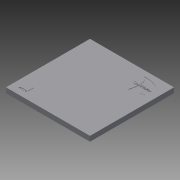
# Autodesk Inventor part: EmbossTest
Saved by Autodesk Inventor 2015 (Build 190159000, 159)
## iProperties
Created: 2014-08-09
Part Number: EmbossTest
Material: Generic
Document SubType Name: Modeling
Designer: Patrick Camilleri
Density: 1 g/cm^3
Appearance: Default
Author: Patrick Camilleri
Autodesk Inventor part; units mm, degrees
(part 1 of 2)
ref_plane "YZ Plane" through (0, 0, 0) normal (1, 0, 0) x (0, 1, 0)
ref_plane "XZ Plane" through (0, 0, 0) normal (0, 1, 0) x (-1, 0, 0)
ref_plane "XY Plane" through (0, 0, 0) normal (0, 0, 1) x (1, 0, 0)
sketch "Sketch1" plane through (0, 0, 0) normal (0, 0, 1) x (1, 0, 0)
  line L0 (-50, 50) -> (50, 50)
  line L1 (50, 50) -> (50, -50)
  line L2 (50, -50) -> (-50, -50)
  line L3 (-50, -50) -> (-50, 50)
  line L4 (-50, 50) -> (50, -50) construction
  line L5 (50, 50) -> (-50, -50) construction
  point P0 (0, 0)
  dimension "d0" = 100
  dimension "d1" = 100
  constraints: 12 end point, 2 midpoint, 2 parallel, 1 horizontal, 1 perpendicular
  measures "d0" distance of L1.end L2.end
  measures "d1" distance of L0.end L1.end
extrude "Extrusion1" add sketch "Sketch1" along normal blind 6
sketch "Sketch2" plane through (0, 0, 6) normal (0, 0, 1) x (1, 0, 0)
  spline S0 degree 3 poles (-34.8118, -41.5172) (-35.008, -41.7253) (-35.2042, -41.9334) (-35.4003, -42.1415) (-35.491, -42.2378) (-35.5355, -42.2383) (-35.6243, -42.1439) (-35.8031, -41.9538) (-35.9823, -41.7641) (-36.1607, -41.5736) (-36.1793, -41.5537) (-36.1936, -41.5297) (-36.2099, -41.5077) (-36.2185, -41.5128) (-36.2271, -41.5179) (-36.2357, -41.523) (-36.2357, -41.9827) (-36.2357, -42.4423) (-36.2357, -42.9059) (-36.4488, -42.9059) (-36.6508, -42.9059) (-36.8568, -42.9059) (-36.8568, -42.1529) (-36.8568, -41.4056) (-36.8568, -40.6466) (-36.6841, -40.6466) (-36.5132, -40.6444) (-36.3424, -40.649) (-36.3174, -40.6497) (-36.29, -40.6795) (-36.269, -40.701) (-36.0168, -40.9595) (-35.7656, -41.219) (-35.4885, -41.5046) (-35.4711, -41.4734) (-35.4606, -41.4412) (-35.4396, -41.4189) (-35.2133, -41.179) (-34.9844, -40.9416) (-34.7587, -40.701) (-34.7199, -40.6596) (-34.6805, -40.6436) (-34.6245, -40.6449) (-34.4757, -40.6483) (-34.3267, -40.646) (-34.1712, -40.646) (-34.1712, -41.4005) (-34.1712, -42.1498) (-34.1712, -42.9054) (-34.3761, -42.9054) (-34.5781, -42.9054) (-34.7897, -42.9054) (-34.7897, -42.4441) (-34.7897, -41.9842) (-34.7897, -41.5243) (-34.797, -41.522) (-34.8044, -41.5196) (-34.8118, -41.5172) knots 0 0 0 0 1 1 1 2 2 2 3 3 3 4 4 4 5 5 5 6 6 6 7 7 7 8 8 8 9 9 9 10 10 10 11 11 11 12 12 12 13 13 13 14 14 14 15 15 15 16 16 16 17 17 17 18 18 18 19 19 19 19
  line L0 (-34.8118, -41.5172) -> (-35.008, -41.7253) construction
  line L1 (-35.008, -41.7253) -> (-35.2042, -41.9334) construction
  line L2 (-35.2042, -41.9334) -> (-35.4003, -42.1415) construction
  line L3 (-35.4003, -42.1415) -> (-35.491, -42.2378) construction
  line L4 (-35.491, -42.2378) -> (-35.5355, -42.2383) construction
  line L5 (-35.5355, -42.2383) -> (-35.6243, -42.1439) construction
  line L6 (-35.6243, -42.1439) -> (-35.8031, -41.9538) construction
  line L7 (-35.8031, -41.9538) -> (-35.9823, -41.7641) construction
  line L8 (-35.9823, -41.7641) -> (-36.1607, -41.5736) construction
  line L9 (-36.1607, -41.5736) -> (-36.1793, -41.5537) construction
  line L10 (-36.1793, -41.5537) -> (-36.1936, -41.5297) construction
  line L11 (-36.1936, -41.5297) -> (-36.2099, -41.5077) construction
  line L12 (-36.2099, -41.5077) -> (-36.2185, -41.5128) construction
  line L13 (-36.2185, -41.5128) -> (-36.2271, -41.5179) construction
  line L14 (-36.2271, -41.5179) -> (-36.2357, -41.523) construction
  line L15 (-36.2357, -41.523) -> (-36.2357, -41.9827) construction
  line L16 (-36.2357, -41.9827) -> (-36.2357, -42.4423) construction
  line L17 (-36.2357, -42.4423) -> (-36.2357, -42.9059) construction
  line L18 (-36.2357, -42.9059) -> (-36.4488, -42.9059) construction
  line L19 (-36.4488, -42.9059) -> (-36.6508, -42.9059) construction
  line L20 (-36.6508, -42.9059) -> (-36.8568, -42.9059) construction
  line L21 (-36.8568, -42.9059) -> (-36.8568, -42.1529) construction
  line L22 (-36.8568, -42.1529) -> (-36.8568, -41.4056) construction
  line L23 (-36.8568, -41.4056) -> (-36.8568, -40.6466) construction
  line L24 (-36.8568, -40.6466) -> (-36.6841, -40.6466) construction
  line L25 (-36.6841, -40.6466) -> (-36.5132, -40.6444) construction
  line L26 (-36.5132, -40.6444) -> (-36.3424, -40.649) construction
  line L27 (-36.3424, -40.649) -> (-36.3174, -40.6497) construction
  line L28 (-36.3174, -40.6497) -> (-36.29, -40.6795) construction
  line L29 (-36.29, -40.6795) -> (-36.269, -40.701) construction
  line L30 (-36.269, -40.701) -> (-36.0168, -40.9595) construction
  line L31 (-36.0168, -40.9595) -> (-35.7656, -41.219) construction
  line L32 (-35.7656, -41.219) -> (-35.4885, -41.5046) construction
  line L33 (-35.4885, -41.5046) -> (-35.4711, -41.4734) construction
  line L34 (-35.4711, -41.4734) -> (-35.4606, -41.4412) construction
  line L35 (-35.4606, -41.4412) -> (-35.4396, -41.4189) construction
  line L36 (-35.4396, -41.4189) -> (-35.2133, -41.179) construction
  line L37 (-35.2133, -41.179) -> (-34.9844, -40.9416) construction
  line L38 (-34.9844, -40.9416) -> (-34.7587, -40.701) construction
  line L39 (-34.7587, -40.701) -> (-34.7199, -40.6596) construction
  line L40 (-34.7199, -40.6596) -> (-34.6805, -40.6436) construction
  line L41 (-34.6805, -40.6436) -> (-34.6245, -40.6449) construction
  line L42 (-34.6245, -40.6449) -> (-34.4757, -40.6483) construction
  line L43 (-34.4757, -40.6483) -> (-34.3267, -40.646) construction
  line L44 (-34.3267, -40.646) -> (-34.1712, -40.646) construction
  line L45 (-34.1712, -40.646) -> (-34.1712, -41.4005) construction
  line L46 (-34.1712, -41.4005) -> (-34.1712, -42.1498) construction
  line L47 (-34.1712, -42.1498) -> (-34.1712, -42.9054) construction
  line L48 (-34.1712, -42.9054) -> (-34.3761, -42.9054) construction
  line L49 (-34.3761, -42.9054) -> (-34.5781, -42.9054) construction
  line L50 (-34.5781, -42.9054) -> (-34.7897, -42.9054) construction
  line L51 (-34.7897, -42.9054) -> (-34.7897, -42.4441) construction
  line L52 (-34.7897, -42.4441) -> (-34.7897, -41.9842) construction
  line L53 (-34.7897, -41.9842) -> (-34.7897, -41.5243) construction
  line L54 (-34.7897, -41.5243) -> (-34.797, -41.522) construction
  line L55 (-34.797, -41.522) -> (-34.8044, -41.5196) construction
  line L56 (-34.8044, -41.5196) -> (-34.8118, -41.5172) construction
  spline S1 degree 3 poles (-39.2287, -40.6616) (-38.7914, -40.6616) (-38.3614, -40.6502) (-37.9325, -40.6665) (-37.7171, -40.6747) (-37.5328, -40.7855) (-37.4045, -40.9677) (-37.2119, -41.2411) (-37.2808, -41.5889) (-37.5615, -41.7698) (-37.6066, -41.7989) (-37.6545, -41.8234) (-37.709, -41.8545) (-37.5451, -41.9467) (-37.4576, -42.0939) (-37.3778, -42.2464) (-37.2652, -42.4612) (-37.1555, -42.6775) (-37.0396, -42.9027) (-37.073, -42.9065) (-37.0944, -42.9111) (-37.1158, -42.9112) (-37.2936, -42.9118) (-37.4714, -42.9093) (-37.6491, -42.9128) (-37.703, -42.9139) (-37.7326, -42.8953) (-37.7552, -42.8482) (-37.8172, -42.7192) (-37.8821, -42.5916) (-37.9469, -42.464) (-37.9819, -42.3951) (-38.0185, -42.3269) (-38.0554, -42.259) (-38.1716, -42.0454) (-38.3477, -41.9527) (-38.601, -41.9994) (-38.6025, -42.0249) (-38.6059, -42.0549) (-38.606, -42.085) (-38.6064, -42.3344) (-38.6078, -42.5839) (-38.6051, -42.8333) (-38.6045, -42.8918) (-38.6202, -42.914) (-38.682, -42.9127) (-38.862, -42.9092) (-39.0422, -42.9115) (-39.2287, -42.9115) (-39.2287, -42.1545) (-39.2287, -41.4055) (-39.2287, -40.6616) knots 0 0 0 0 1 1 1 2 2 2 3 3 3 4 4 4 5 5 5 6 6 6 7 7 7 8 8 8 9 9 9 10 10 10 11 11 11 12 12 12 13 13 13 14 14 14 15 15 15 16 16 16 17 17 17 17
  line L57 (-39.2287, -40.6616) -> (-38.7914, -40.6616) construction
  line L58 (-38.7914, -40.6616) -> (-38.3614, -40.6502) construction
  line L59 (-38.3614, -40.6502) -> (-37.9325, -40.6665) construction
  line L60 (-37.9325, -40.6665) -> (-37.7171, -40.6747) construction
  line L61 (-37.7171, -40.6747) -> (-37.5328, -40.7855) construction
  line L62 (-37.5328, -40.7855) -> (-37.4045, -40.9677) construction
  line L63 (-37.4045, -40.9677) -> (-37.2119, -41.2411) construction
  line L64 (-37.2119, -41.2411) -> (-37.2808, -41.5889) construction
  line L65 (-37.2808, -41.5889) -> (-37.5615, -41.7698) construction
  line L66 (-37.5615, -41.7698) -> (-37.6066, -41.7989) construction
  line L67 (-37.6066, -41.7989) -> (-37.6545, -41.8234) construction
  line L68 (-37.6545, -41.8234) -> (-37.709, -41.8545) construction
  line L69 (-37.709, -41.8545) -> (-37.5451, -41.9467) construction
  line L70 (-37.5451, -41.9467) -> (-37.4576, -42.0939) construction
  line L71 (-37.4576, -42.0939) -> (-37.3778, -42.2464) construction
  line L72 (-37.3778, -42.2464) -> (-37.2652, -42.4612) construction
  line L73 (-37.2652, -42.4612) -> (-37.1555, -42.6775) construction
  line L74 (-37.1555, -42.6775) -> (-37.0396, -42.9027) construction
  line L75 (-37.0396, -42.9027) -> (-37.073, -42.9065) construction
  line L76 (-37.073, -42.9065) -> (-37.0944, -42.9111) construction
  line L77 (-37.0944, -42.9111) -> (-37.1158, -42.9112) construction
  line L78 (-37.1158, -42.9112) -> (-37.2936, -42.9118) construction
  line L79 (-37.2936, -42.9118) -> (-37.4714, -42.9093) construction
  line L80 (-37.4714, -42.9093) -> (-37.6491, -42.9128) construction
  line L81 (-37.6491, -42.9128) -> (-37.703, -42.9139) construction
  line L82 (-37.703, -42.9139) -> (-37.7326, -42.8953) construction
  line L83 (-37.7326, -42.8953) -> (-37.7552, -42.8482) construction
  line L84 (-37.7552, -42.8482) -> (-37.8172, -42.7192) construction
  line L85 (-37.8172, -42.7192) -> (-37.8821, -42.5916) construction
  line L86 (-37.8821, -42.5916) -> (-37.9469, -42.464) construction
  line L87 (-37.9469, -42.464) -> (-37.9819, -42.3951) construction
  line L88 (-37.9819, -42.3951) -> (-38.0185, -42.3269) construction
  line L89 (-38.0185, -42.3269) -> (-38.0554, -42.259) construction
  line L90 (-38.0554, -42.259) -> (-38.1716, -42.0454) construction
  line L91 (-38.1716, -42.0454) -> (-38.3477, -41.9527) construction
  line L92 (-38.3477, -41.9527) -> (-38.601, -41.9994) construction
  line L93 (-38.601, -41.9994) -> (-38.6025, -42.0249) construction
  line L94 (-38.6025, -42.0249) -> (-38.6059, -42.0549) construction
  line L95 (-38.6059, -42.0549) -> (-38.606, -42.085) construction
  line L96 (-38.606, -42.085) -> (-38.6064, -42.3344) construction
  line L97 (-38.6064, -42.3344) -> (-38.6078, -42.5839) construction
  line L98 (-38.6078, -42.5839) -> (-38.6051, -42.8333) construction
  line L99 (-38.6051, -42.8333) -> (-38.6045, -42.8918) construction
  line L100 (-38.6045, -42.8918) -> (-38.6202, -42.914) construction
  line L101 (-38.6202, -42.914) -> (-38.682, -42.9127) construction
  line L102 (-38.682, -42.9127) -> (-38.862, -42.9092) construction
  line L103 (-38.862, -42.9092) -> (-39.0422, -42.9115) construction
  line L104 (-39.0422, -42.9115) -> (-39.2287, -42.9115) construction
  line L105 (-39.2287, -42.9115) -> (-39.2287, -42.1545) construction
  line L106 (-39.2287, -42.1545) -> (-39.2287, -41.4055) construction
  line L107 (-39.2287, -41.4055) -> (-39.2287, -40.6616) construction
  spline S2 degree 3 poles (-38.6, -41.0537) (-38.6, -41.2363) (-38.6, -41.4025) (-38.6, -41.5842) (-38.4373, -41.5746) (-38.2798, -41.5763) (-38.1261, -41.553) (-37.9994, -41.5338) (-37.9376, -41.4371) (-37.9393, -41.3124) (-37.9411, -41.1891) (-38.0091, -41.0963) (-38.1362, -41.0804) (-38.2878, -41.0614) (-38.4418, -41.0619) (-38.6, -41.0537) knots 0 0 0 0 1 1 1 2 2 2 3 3 3 4 4 4 5 5 5 5
  line L108 (-38.6, -41.0537) -> (-38.6, -41.2363) construction
  line L109 (-38.6, -41.2363) -> (-38.6, -41.4025) construction
  line L110 (-38.6, -41.4025) -> (-38.6, -41.5842) construction
  line L111 (-38.6, -41.5842) -> (-38.4373, -41.5746) construction
  line L112 (-38.4373, -41.5746) -> (-38.2798, -41.5763) construction
  line L113 (-38.2798, -41.5763) -> (-38.1261, -41.553) construction
  line L114 (-38.1261, -41.553) -> (-37.9994, -41.5338) construction
  line L115 (-37.9994, -41.5338) -> (-37.9376, -41.4371) construction
  line L116 (-37.9376, -41.4371) -> (-37.9393, -41.3124) construction
  line L117 (-37.9393, -41.3124) -> (-37.9411, -41.1891) construction
  line L118 (-37.9411, -41.1891) -> (-38.0091, -41.0963) construction
  line L119 (-38.0091, -41.0963) -> (-38.1362, -41.0804) construction
  line L120 (-38.1362, -41.0804) -> (-38.2878, -41.0614) construction
  line L121 (-38.2878, -41.0614) -> (-38.4418, -41.0619) construction
  line L122 (-38.4418, -41.0619) -> (-38.6, -41.0537) construction
  spline S3 degree 3 poles (-39.3868, -42.9109) (-39.605, -42.9109) (-39.813, -42.9124) (-40.0209, -42.9084) (-40.0397, -42.908) (-40.0643, -42.8756) (-40.0752, -42.8528) (-40.126, -42.7469) (-40.1755, -42.6404) (-40.22, -42.5319) (-40.2419, -42.4784) (-40.2731, -42.4621) (-40.3302, -42.4626) (-40.6513, -42.4656) (-40.9724, -42.4654) (-41.2935, -42.4629) (-41.3528, -42.4624) (-41.3864, -42.4767) (-41.408, -42.5368) (-41.4466, -42.6444) (-41.4937, -42.7491) (-41.5418, -42.8529) (-41.5528, -42.8767) (-41.5817, -42.9083) (-41.6029, -42.9088) (-41.8028, -42.913) (-42.0029, -42.9113) (-42.2145, -42.9113) (-42.1997, -42.873) (-42.1901, -42.8444) (-42.1779, -42.817) (-41.8681, -42.1183) (-41.5576, -41.42) (-41.2493, -40.7208) (-41.2256, -40.6671) (-41.1998, -40.6427) (-41.1367, -40.6443) (-40.9419, -40.6492) (-40.7468, -40.6473) (-40.5519, -40.6451) (-40.5067, -40.6447) (-40.4803, -40.6557) (-40.4591, -40.6996) (-40.11, -41.4179) (-39.7589, -42.1353) (-39.4085, -42.853) (-39.4015, -42.8675) (-39.3971, -42.8832) (-39.3868, -42.9109) knots 0 0 0 0 1 1 1 2 2 2 3 3 3 4 4 4 5 5 5 6 6 6 7 7 7 8 8 8 9 9 9 10 10 10 11 11 11 12 12 12 13 13 13 14 14 14 15 15 15 16 16 16 16
  line L123 (-39.3868, -42.9109) -> (-39.605, -42.9109) construction
  line L124 (-39.605, -42.9109) -> (-39.813, -42.9124) construction
  line L125 (-39.813, -42.9124) -> (-40.0209, -42.9084) construction
  line L126 (-40.0209, -42.9084) -> (-40.0397, -42.908) construction
  line L127 (-40.0397, -42.908) -> (-40.0643, -42.8756) construction
  line L128 (-40.0643, -42.8756) -> (-40.0752, -42.8528) construction
  line L129 (-40.0752, -42.8528) -> (-40.126, -42.7469) construction
  line L130 (-40.126, -42.7469) -> (-40.1755, -42.6404) construction
  line L131 (-40.1755, -42.6404) -> (-40.22, -42.5319) construction
  line L132 (-40.22, -42.5319) -> (-40.2419, -42.4784) construction
  line L133 (-40.2419, -42.4784) -> (-40.2731, -42.4621) construction
  line L134 (-40.2731, -42.4621) -> (-40.3302, -42.4626) construction
  line L135 (-40.3302, -42.4626) -> (-40.6513, -42.4656) construction
  line L136 (-40.6513, -42.4656) -> (-40.9724, -42.4654) construction
  line L137 (-40.9724, -42.4654) -> (-41.2935, -42.4629) construction
  line L138 (-41.2935, -42.4629) -> (-41.3528, -42.4624) construction
  line L139 (-41.3528, -42.4624) -> (-41.3864, -42.4767) construction
  line L140 (-41.3864, -42.4767) -> (-41.408, -42.5368) construction
  line L141 (-41.408, -42.5368) -> (-41.4466, -42.6444) construction
  line L142 (-41.4466, -42.6444) -> (-41.4937, -42.7491) construction
  line L143 (-41.4937, -42.7491) -> (-41.5418, -42.8529) construction
  line L144 (-41.5418, -42.8529) -> (-41.5528, -42.8767) construction
  line L145 (-41.5528, -42.8767) -> (-41.5817, -42.9083) construction
  line L146 (-41.5817, -42.9083) -> (-41.6029, -42.9088) construction
  line L147 (-41.6029, -42.9088) -> (-41.8028, -42.913) construction
  line L148 (-41.8028, -42.913) -> (-42.0029, -42.9113) construction
  line L149 (-42.0029, -42.9113) -> (-42.2145, -42.9113) construction
  line L150 (-42.2145, -42.9113) -> (-42.1997, -42.873) construction
  line L151 (-42.1997, -42.873) -> (-42.1901, -42.8444) construction
  line L152 (-42.1901, -42.8444) -> (-42.1779, -42.817) construction
  line L153 (-42.1779, -42.817) -> (-41.8681, -42.1183) construction
  line L154 (-41.8681, -42.1183) -> (-41.5576, -41.42) construction
  line L155 (-41.5576, -41.42) -> (-41.2493, -40.7208) construction
  line L156 (-41.2493, -40.7208) -> (-41.2256, -40.6671) construction
  line L157 (-41.2256, -40.6671) -> (-41.1998, -40.6427) construction
  line L158 (-41.1998, -40.6427) -> (-41.1367, -40.6443) construction
  line L159 (-41.1367, -40.6443) -> (-40.9419, -40.6492) construction
  line L160 (-40.9419, -40.6492) -> (-40.7468, -40.6473) construction
  line L161 (-40.7468, -40.6473) -> (-40.5519, -40.6451) construction
  line L162 (-40.5519, -40.6451) -> (-40.5067, -40.6447) construction
  line L163 (-40.5067, -40.6447) -> (-40.4803, -40.6557) construction
  line L164 (-40.4803, -40.6557) -> (-40.4591, -40.6996) construction
  line L165 (-40.4591, -40.6996) -> (-40.11, -41.4179) construction
  line L166 (-40.11, -41.4179) -> (-39.7589, -42.1353) construction
  line L167 (-39.7589, -42.1353) -> (-39.4085, -42.853) construction
  line L168 (-39.4085, -42.853) -> (-39.4015, -42.8675) construction
  line L169 (-39.4015, -42.8675) -> (-39.3971, -42.8832) construction
  line L170 (-39.3971, -42.8832) -> (-39.3868, -42.9109) construction
  spline S4 degree 3 poles (-40.8503, -41.1882) (-40.9747, -41.4892) (-41.0919, -41.7726) (-41.2123, -42.0639) (-40.9517, -42.0639) (-40.7052, -42.0639) (-40.4452, -42.0639) (-40.5801, -41.7725) (-40.7104, -41.4908) (-40.8503, -41.1882) knots 0 0 0 0 1 1 1 2 2 2 3 3 3 3
  line L171 (-40.8503, -41.1882) -> (-40.9747, -41.4892) construction
  line L172 (-40.9747, -41.4892) -> (-41.0919, -41.7726) construction
  line L173 (-41.0919, -41.7726) -> (-41.2123, -42.0639) construction
  line L174 (-41.2123, -42.0639) -> (-40.9517, -42.0639) construction
  line L175 (-40.9517, -42.0639) -> (-40.7052, -42.0639) construction
  line L176 (-40.7052, -42.0639) -> (-40.4452, -42.0639) construction
  line L177 (-40.4452, -42.0639) -> (-40.5801, -41.7725) construction
  line L178 (-40.5801, -41.7725) -> (-40.7104, -41.4908) construction
  line L179 (-40.7104, -41.4908) -> (-40.8503, -41.1882) construction
  spline S5 degree 3 poles (-33.8681, -41.7853) (-33.4616, -41.7853) (-33.0617, -41.7853) (-32.6568, -41.7853) (-32.6568, -42.1521) (-32.6568, -42.5147) (-32.6568, -42.8858) (-33.0581, -42.8858) (-33.4597, -42.8858) (-33.8681, -42.8858) (-33.8681, -42.5215) (-33.8681, -42.1567) (-33.8681, -41.7853) knots 0 0 0 0 1 1 1 2 2 2 3 3 3 4 4 4 4
  line L180 (-33.8681, -41.7853) -> (-33.4616, -41.7853) construction
  line L181 (-33.4616, -41.7853) -> (-33.0617, -41.7853) construction
  line L182 (-33.0617, -41.7853) -> (-32.6568, -41.7853) construction
  line L183 (-32.6568, -41.7853) -> (-32.6568, -42.1521) construction
  line L184 (-32.6568, -42.1521) -> (-32.6568, -42.5147) construction
  line L185 (-32.6568, -42.5147) -> (-32.6568, -42.8858) construction
  line L186 (-32.6568, -42.8858) -> (-33.0581, -42.8858) construction
  line L187 (-33.0581, -42.8858) -> (-33.4597, -42.8858) construction
  line L188 (-33.4597, -42.8858) -> (-33.8681, -42.8858) construction
  line L189 (-33.8681, -42.8858) -> (-33.8681, -42.5215) construction
  line L190 (-33.8681, -42.5215) -> (-33.8681, -42.1567) construction
  line L191 (-33.8681, -42.1567) -> (-33.8681, -41.7853) construction
  spline S6 degree 3 poles (-33.7217, -38.9912) (-33.7217, -38.9387) (-33.7217, -38.8916) (-33.7217, -38.8362) (-33.3924, -38.7709) (-33.0623, -38.7054) (-32.7322, -38.64) (-32.7316, -38.6337) (-32.731, -38.6274) (-32.7304, -38.6211) (-32.8416, -38.5965) (-32.9527, -38.5713) (-33.0641, -38.5474) (-33.2515, -38.507) (-33.4382, -38.4621) (-33.6271, -38.4302) (-33.7109, -38.416) (-33.7412, -38.3833) (-33.728, -38.3024) (-33.724, -38.2775) (-33.7274, -38.2514) (-33.7274, -38.2181) (-33.3898, -38.1562) (-33.0567, -38.095) (-32.7235, -38.0338) (-32.7237, -38.0281) (-32.7239, -38.0224) (-32.7241, -38.0166) (-33.0236, -37.9482) (-33.3232, -37.88) (-33.6227, -37.8113) (-33.7406, -37.7842) (-33.7404, -37.7836) (-33.7165, -37.6482) (-33.5086, -37.7002) (-33.3012, -37.7521) (-33.0938, -37.8038) (-32.9245, -37.8459) (-32.7559, -37.8916) (-32.5852, -37.9279) (-32.5122, -37.9435) (-32.5195, -37.9881) (-32.5163, -38.0407) (-32.5128, -38.099) (-32.5415, -38.1107) (-32.5906, -38.1201) (-32.897, -38.1788) (-33.2027, -38.2407) (-33.5087, -38.3017) (-33.5236, -38.3047) (-33.5381, -38.3095) (-33.553, -38.3306) (-33.2108, -38.4036) (-32.8687, -38.4766) (-32.5301, -38.5489) (-32.5251, -38.5595) (-32.5211, -38.5644) (-32.5205, -38.5698) (-32.5041, -38.7211) (-32.5042, -38.7208) (-32.6525, -38.7541) (-32.9932, -38.8305) (-33.3338, -38.9071) (-33.6745, -38.9835) (-33.6879, -38.9865) (-33.7017, -38.988) (-33.7217, -38.9912) knots 0 0 0 0 1 1 1 2 2 2 3 3 3 4 4 4 5 5 5 6 6 6 7 7 7 8 8 8 9 9 9 10 10 10 11 11 11 12 12 12 13 13 13 14 14 14 15 15 15 16 16 16 17 17 17 18 18 18 19 19 19 20 20 20 21 21 21 22 22 22 22
  line L192 (-33.7217, -38.9912) -> (-33.7217, -38.9387) construction
  line L193 (-33.7217, -38.9387) -> (-33.7217, -38.8916) construction
  line L194 (-33.7217, -38.8916) -> (-33.7217, -38.8362) construction
  line L195 (-33.7217, -38.8362) -> (-33.3924, -38.7709) construction
  line L196 (-33.3924, -38.7709) -> (-33.0623, -38.7054) construction
  line L197 (-33.0623, -38.7054) -> (-32.7322, -38.64) construction
  line L198 (-32.7322, -38.64) -> (-32.7316, -38.6337) construction
  line L199 (-32.7316, -38.6337) -> (-32.731, -38.6274) construction
  line L200 (-32.731, -38.6274) -> (-32.7304, -38.6211) construction
  line L201 (-32.7304, -38.6211) -> (-32.8416, -38.5965) construction
  line L202 (-32.8416, -38.5965) -> (-32.9527, -38.5713) construction
  line L203 (-32.9527, -38.5713) -> (-33.0641, -38.5474) construction
  line L204 (-33.0641, -38.5474) -> (-33.2515, -38.507) construction
  line L205 (-33.2515, -38.507) -> (-33.4382, -38.4621) construction
  line L206 (-33.4382, -38.4621) -> (-33.6271, -38.4302) construction
  line L207 (-33.6271, -38.4302) -> (-33.7109, -38.416) construction
  line L208 (-33.7109, -38.416) -> (-33.7412, -38.3833) construction
  line L209 (-33.7412, -38.3833) -> (-33.728, -38.3024) construction
  line L210 (-33.728, -38.3024) -> (-33.724, -38.2775) construction
  line L211 (-33.724, -38.2775) -> (-33.7274, -38.2514) construction
  line L212 (-33.7274, -38.2514) -> (-33.7274, -38.2181) construction
  line L213 (-33.7274, -38.2181) -> (-33.3898, -38.1562) construction
  line L214 (-33.3898, -38.1562) -> (-33.0567, -38.095) construction
  line L215 (-33.0567, -38.095) -> (-32.7235, -38.0338) construction
  line L216 (-32.7235, -38.0338) -> (-32.7237, -38.0281) construction
  line L217 (-32.7237, -38.0281) -> (-32.7239, -38.0224) construction
  line L218 (-32.7239, -38.0224) -> (-32.7241, -38.0166) construction
  line L219 (-32.7241, -38.0166) -> (-33.0236, -37.9482) construction
  line L220 (-33.0236, -37.9482) -> (-33.3232, -37.88) construction
  line L221 (-33.3232, -37.88) -> (-33.6227, -37.8113) construction
  line L222 (-33.6227, -37.8113) -> (-33.7406, -37.7842) construction
  line L223 (-33.7406, -37.7842) -> (-33.7404, -37.7836) construction
  line L224 (-33.7404, -37.7836) -> (-33.7165, -37.6482) construction
  line L225 (-33.7165, -37.6482) -> (-33.5086, -37.7002) construction
  line L226 (-33.5086, -37.7002) -> (-33.3012, -37.7521) construction
  line L227 (-33.3012, -37.7521) -> (-33.0938, -37.8038) construction
  line L228 (-33.0938, -37.8038) -> (-32.9245, -37.8459) construction
  line L229 (-32.9245, -37.8459) -> (-32.7559, -37.8916) construction
  line L230 (-32.7559, -37.8916) -> (-32.5852, -37.9279) construction
  line L231 (-32.5852, -37.9279) -> (-32.5122, -37.9435) construction
  line L232 (-32.5122, -37.9435) -> (-32.5195, -37.9881) construction
  line L233 (-32.5195, -37.9881) -> (-32.5163, -38.0407) construction
  line L234 (-32.5163, -38.0407) -> (-32.5128, -38.099) construction
  line L235 (-32.5128, -38.099) -> (-32.5415, -38.1107) construction
  line L236 (-32.5415, -38.1107) -> (-32.5906, -38.1201) construction
  line L237 (-32.5906, -38.1201) -> (-32.897, -38.1788) construction
  line L238 (-32.897, -38.1788) -> (-33.2027, -38.2407) construction
  line L239 (-33.2027, -38.2407) -> (-33.5087, -38.3017) construction
  line L240 (-33.5087, -38.3017) -> (-33.5236, -38.3047) construction
  line L241 (-33.5236, -38.3047) -> (-33.5381, -38.3095) construction
  line L242 (-33.5381, -38.3095) -> (-33.553, -38.3306) construction
  line L243 (-33.553, -38.3306) -> (-33.2108, -38.4036) construction
  line L244 (-33.2108, -38.4036) -> (-32.8687, -38.4766) construction
  line L245 (-32.8687, -38.4766) -> (-32.5301, -38.5489) construction
  line L246 (-32.5301, -38.5489) -> (-32.5251, -38.5595) construction
  line L247 (-32.5251, -38.5595) -> (-32.5211, -38.5644) construction
  line L248 (-32.5211, -38.5644) -> (-32.5205, -38.5698) construction
  line L249 (-32.5205, -38.5698) -> (-32.5041, -38.7211) construction
  line L250 (-32.5041, -38.7211) -> (-32.5042, -38.7208) construction
  line L251 (-32.5042, -38.7208) -> (-32.6525, -38.7541) construction
  line L252 (-32.6525, -38.7541) -> (-32.9932, -38.8305) construction
  line L253 (-32.9932, -38.8305) -> (-33.3338, -38.9071) construction
  line L254 (-33.3338, -38.9071) -> (-33.6745, -38.9835) construction
  line L255 (-33.6745, -38.9835) -> (-33.6879, -38.9865) construction
  line L256 (-33.6879, -38.9865) -> (-33.7017, -38.988) construction
  line L257 (-33.7017, -38.988) -> (-33.7217, -38.9912) construction
  spline S7 degree 3 poles (-33.7147, -35.2257) (-33.7147, -35.0772) (-33.7216, -34.9371) (-33.7126, -34.7981) (-33.7053, -34.6847) (-33.6212, -34.6185) (-33.5216, -34.5885) (-33.3183, -34.5272) (-33.1082, -34.545) (-32.8999, -34.5575) (-32.8439, -34.5609) (-32.7864, -34.5714) (-32.7335, -34.5897) (-32.5911, -34.6387) (-32.5181, -34.7452) (-32.5179, -34.8936) (-32.5177, -34.9968) (-32.5186, -35.1) (-32.5194, -35.2033) (-32.5194, -35.2085) (-32.5232, -35.2138) (-32.5279, -35.2257) (-32.922, -35.2257) (-33.3187, -35.2257) (-33.7147, -35.2257) knots 0 0 0 0 1 1 1 2 2 2 3 3 3 4 4 4 5 5 5 6 6 6 7 7 7 8 8 8 8
  line L258 (-33.7147, -35.2257) -> (-33.7147, -35.0772) construction
  line L259 (-33.7147, -35.0772) -> (-33.7216, -34.9371) construction
  line L260 (-33.7216, -34.9371) -> (-33.7126, -34.7981) construction
  line L261 (-33.7126, -34.7981) -> (-33.7053, -34.6847) construction
  line L262 (-33.7053, -34.6847) -> (-33.6212, -34.6185) construction
  line L263 (-33.6212, -34.6185) -> (-33.5216, -34.5885) construction
  line L264 (-33.5216, -34.5885) -> (-33.3183, -34.5272) construction
  line L265 (-33.3183, -34.5272) -> (-33.1082, -34.545) construction
  line L266 (-33.1082, -34.545) -> (-32.8999, -34.5575) construction
  line L267 (-32.8999, -34.5575) -> (-32.8439, -34.5609) construction
  line L268 (-32.8439, -34.5609) -> (-32.7864, -34.5714) construction
  line L269 (-32.7864, -34.5714) -> (-32.7335, -34.5897) construction
  line L270 (-32.7335, -34.5897) -> (-32.5911, -34.6387) construction
  line L271 (-32.5911, -34.6387) -> (-32.5181, -34.7452) construction
  line L272 (-32.5181, -34.7452) -> (-32.5179, -34.8936) construction
  line L273 (-32.5179, -34.8936) -> (-32.5177, -34.9968) construction
  line L274 (-32.5177, -34.9968) -> (-32.5186, -35.1) construction
  line L275 (-32.5186, -35.1) -> (-32.5194, -35.2033) construction
  line L276 (-32.5194, -35.2033) -> (-32.5194, -35.2085) construction
  line L277 (-32.5194, -35.2085) -> (-32.5232, -35.2138) construction
  line L278 (-32.5232, -35.2138) -> (-32.5279, -35.2257) construction
  line L279 (-32.5279, -35.2257) -> (-32.922, -35.2257) construction
  line L280 (-32.922, -35.2257) -> (-33.3187, -35.2257) construction
  line L281 (-33.3187, -35.2257) -> (-33.7147, -35.2257) construction
  spline S8 degree 3 poles (-32.6481, -35.0843) (-32.6481, -35.0388) (-32.6499, -35.0019) (-32.6478, -34.9651) (-32.6391, -34.8163) (-32.7076, -34.7085) (-32.8525, -34.7051) (-33.0483, -34.7005) (-33.2448, -34.6987) (-33.4401, -34.7112) (-33.5222, -34.7164) (-33.5858, -34.7798) (-33.5945, -34.8708) (-33.6011, -34.9405) (-33.5958, -35.0114) (-33.5958, -35.0843) (-33.2779, -35.0843) (-32.9693, -35.0843) (-32.6481, -35.0843) knots 0 0 0 0 1 1 1 2 2 2 3 3 3 4 4 4 5 5 5 6 6 6 6
  line L282 (-32.6481, -35.0843) -> (-32.6481, -35.0388) construction
  line L283 (-32.6481, -35.0388) -> (-32.6499, -35.0019) construction
  line L284 (-32.6499, -35.0019) -> (-32.6478, -34.9651) construction
  line L285 (-32.6478, -34.9651) -> (-32.6391, -34.8163) construction
  line L286 (-32.6391, -34.8163) -> (-32.7076, -34.7085) construction
  line L287 (-32.7076, -34.7085) -> (-32.8525, -34.7051) construction
  line L288 (-32.8525, -34.7051) -> (-33.0483, -34.7005) construction
  line L289 (-33.0483, -34.7005) -> (-33.2448, -34.6987) construction
  line L290 (-33.2448, -34.6987) -> (-33.4401, -34.7112) construction
  line L291 (-33.4401, -34.7112) -> (-33.5222, -34.7164) construction
  line L292 (-33.5222, -34.7164) -> (-33.5858, -34.7798) construction
  line L293 (-33.5858, -34.7798) -> (-33.5945, -34.8708) construction
  line L294 (-33.5945, -34.8708) -> (-33.6011, -34.9405) construction
  line L295 (-33.6011, -34.9405) -> (-33.5958, -35.0114) construction
  line L296 (-33.5958, -35.0114) -> (-33.5958, -35.0843) construction
  line L297 (-33.5958, -35.0843) -> (-33.2779, -35.0843) construction
  line L298 (-33.2779, -35.0843) -> (-32.9693, -35.0843) construction
  line L299 (-32.9693, -35.0843) -> (-32.6481, -35.0843) construction
  spline S9 degree 3 poles (-32.5242, -36.1511) (-32.5077, -36.3021) (-32.5077, -36.3014) (-32.6514, -36.3105) (-32.7453, -36.3164) (-32.8401, -36.3187) (-32.9327, -36.3333) (-33.0313, -36.3489) (-33.0732, -36.4053) (-33.076, -36.5048) (-33.0774, -36.5529) (-33.0763, -36.6009) (-33.0763, -36.6593) (-32.8882, -36.6593) (-32.7089, -36.6593) (-32.5238, -36.6593) (-32.5238, -36.7109) (-32.5238, -36.7522) (-32.5238, -36.7992) (-32.923, -36.7992) (-33.3197, -36.7992) (-33.7249, -36.7992) (-33.7249, -36.6543) (-33.732, -36.5112) (-33.7224, -36.3693) (-33.7156, -36.2697) (-33.6217, -36.189) (-33.5261, -36.1683) (-33.3919, -36.1394) (-33.2722, -36.1529) (-33.183, -36.2707) (-33.1692, -36.2888) (-33.159, -36.3096) (-33.1416, -36.3382) (-33.1078, -36.2014) (-33.0053, -36.1892) (-32.8935, -36.184) (-32.7719, -36.1782) (-32.6509, -36.1628) (-32.5242, -36.1511) knots 0 0 0 0 1 1 1 2 2 2 3 3 3 4 4 4 5 5 5 6 6 6 7 7 7 8 8 8 9 9 9 10 10 10 11 11 11 12 12 12 13 13 13 13
  line L300 (-32.5242, -36.1511) -> (-32.5077, -36.3021) construction
  line L301 (-32.5077, -36.3021) -> (-32.5077, -36.3014) construction
  line L302 (-32.5077, -36.3014) -> (-32.6514, -36.3105) construction
  line L303 (-32.6514, -36.3105) -> (-32.7453, -36.3164) construction
  line L304 (-32.7453, -36.3164) -> (-32.8401, -36.3187) construction
  line L305 (-32.8401, -36.3187) -> (-32.9327, -36.3333) construction
  line L306 (-32.9327, -36.3333) -> (-33.0313, -36.3489) construction
  line L307 (-33.0313, -36.3489) -> (-33.0732, -36.4053) construction
  line L308 (-33.0732, -36.4053) -> (-33.076, -36.5048) construction
  line L309 (-33.076, -36.5048) -> (-33.0774, -36.5529) construction
  line L310 (-33.0774, -36.5529) -> (-33.0763, -36.6009) construction
  line L311 (-33.0763, -36.6009) -> (-33.0763, -36.6593) construction
  line L312 (-33.0763, -36.6593) -> (-32.8882, -36.6593) construction
  line L313 (-32.8882, -36.6593) -> (-32.7089, -36.6593) construction
  line L314 (-32.7089, -36.6593) -> (-32.5238, -36.6593) construction
  line L315 (-32.5238, -36.6593) -> (-32.5238, -36.7109) construction
  line L316 (-32.5238, -36.7109) -> (-32.5238, -36.7522) construction
  line L317 (-32.5238, -36.7522) -> (-32.5238, -36.7992) construction
  line L318 (-32.5238, -36.7992) -> (-32.923, -36.7992) construction
  line L319 (-32.923, -36.7992) -> (-33.3197, -36.7992) construction
  line L320 (-33.3197, -36.7992) -> (-33.7249, -36.7992) construction
  line L321 (-33.7249, -36.7992) -> (-33.7249, -36.6543) construction
  line L322 (-33.7249, -36.6543) -> (-33.732, -36.5112) construction
  line L323 (-33.732, -36.5112) -> (-33.7224, -36.3693) construction
  line L324 (-33.7224, -36.3693) -> (-33.7156, -36.2697) construction
  line L325 (-33.7156, -36.2697) -> (-33.6217, -36.189) construction
  line L326 (-33.6217, -36.189) -> (-33.5261, -36.1683) construction
  line L327 (-33.5261, -36.1683) -> (-33.3919, -36.1394) construction
  line L328 (-33.3919, -36.1394) -> (-33.2722, -36.1529) construction
  line L329 (-33.2722, -36.1529) -> (-33.183, -36.2707) construction
  line L330 (-33.183, -36.2707) -> (-33.1692, -36.2888) construction
  line L331 (-33.1692, -36.2888) -> (-33.159, -36.3096) construction
  line L332 (-33.159, -36.3096) -> (-33.1416, -36.3382) construction
  line L333 (-33.1416, -36.3382) -> (-33.1078, -36.2014) construction
  line L334 (-33.1078, -36.2014) -> (-33.0053, -36.1892) construction
  line L335 (-33.0053, -36.1892) -> (-32.8935, -36.184) construction
  line L336 (-32.8935, -36.184) -> (-32.7719, -36.1782) construction
  line L337 (-32.7719, -36.1782) -> (-32.6509, -36.1628) construction
  line L338 (-32.6509, -36.1628) -> (-32.5242, -36.1511) construction
  spline S10 degree 3 poles (-33.5999, -36.6554) (-33.4625, -36.6554) (-33.3354, -36.6554) (-33.1981, -36.6554) (-33.219, -36.5422) (-33.1564, -36.4157) (-33.2762, -36.3358) (-33.3574, -36.2817) (-33.4518, -36.276) (-33.5324, -36.3352) (-33.6467, -36.4192) (-33.5817, -36.5436) (-33.5999, -36.6554) knots 0 0 0 0 1 1 1 2 2 2 3 3 3 4 4 4 4
  line L339 (-33.5999, -36.6554) -> (-33.4625, -36.6554) construction
  line L340 (-33.4625, -36.6554) -> (-33.3354, -36.6554) construction
  line L341 (-33.3354, -36.6554) -> (-33.1981, -36.6554) construction
  line L342 (-33.1981, -36.6554) -> (-33.219, -36.5422) construction
  line L343 (-33.219, -36.5422) -> (-33.1564, -36.4157) construction
  line L344 (-33.1564, -36.4157) -> (-33.2762, -36.3358) construction
  line L345 (-33.2762, -36.3358) -> (-33.3574, -36.2817) construction
  line L346 (-33.3574, -36.2817) -> (-33.4518, -36.276) construction
  line L347 (-33.4518, -36.276) -> (-33.5324, -36.3352) construction
  line L348 (-33.5324, -36.3352) -> (-33.6467, -36.4192) construction
  line L349 (-33.6467, -36.4192) -> (-33.5817, -36.5436) construction
  line L350 (-33.5817, -36.5436) -> (-33.5999, -36.6554) construction
  spline S11 degree 3 poles (-33.1276, -39.7943) (-33.2526, -39.7876) (-33.3653, -39.7917) (-33.4744, -39.7737) (-33.78, -39.7233) (-33.8314, -39.4007) (-33.6717, -39.2103) (-33.6185, -39.1469) (-33.5084, -39.104) (-33.4224, -39.1008) (-33.1952, -39.0924) (-32.9649, -39.0952) (-32.7397, -39.1233) (-32.5448, -39.1477) (-32.4793, -39.2669) (-32.4883, -39.4931) (-32.494, -39.6364) (-32.6002, -39.749) (-32.7652, -39.7702) (-32.8894, -39.7861) (-33.0155, -39.7874) (-33.1276, -39.7943) knots 0 0 0 0 1 1 1 2 2 2 3 3 3 4 4 4 5 5 5 6 6 6 7 7 7 7
  line L351 (-33.1276, -39.7943) -> (-33.2526, -39.7876) construction
  line L352 (-33.2526, -39.7876) -> (-33.3653, -39.7917) construction
  line L353 (-33.3653, -39.7917) -> (-33.4744, -39.7737) construction
  line L354 (-33.4744, -39.7737) -> (-33.78, -39.7233) construction
  line L355 (-33.78, -39.7233) -> (-33.8314, -39.4007) construction
  line L356 (-33.8314, -39.4007) -> (-33.6717, -39.2103) construction
  line L357 (-33.6717, -39.2103) -> (-33.6185, -39.1469) construction
  line L358 (-33.6185, -39.1469) -> (-33.5084, -39.104) construction
  line L359 (-33.5084, -39.104) -> (-33.4224, -39.1008) construction
  line L360 (-33.4224, -39.1008) -> (-33.1952, -39.0924) construction
  line L361 (-33.1952, -39.0924) -> (-32.9649, -39.0952) construction
  line L362 (-32.9649, -39.0952) -> (-32.7397, -39.1233) construction
  line L363 (-32.7397, -39.1233) -> (-32.5448, -39.1477) construction
  line L364 (-32.5448, -39.1477) -> (-32.4793, -39.2669) construction
  line L365 (-32.4793, -39.2669) -> (-32.4883, -39.4931) construction
  line L366 (-32.4883, -39.4931) -> (-32.494, -39.6364) construction
  line L367 (-32.494, -39.6364) -> (-32.6002, -39.749) construction
  line L368 (-32.6002, -39.749) -> (-32.7652, -39.7702) construction
  line L369 (-32.7652, -39.7702) -> (-32.8894, -39.7861) construction
  line L370 (-32.8894, -39.7861) -> (-33.0155, -39.7874) construction
  line L371 (-33.0155, -39.7874) -> (-33.1276, -39.7943) construction
  spline S12 degree 3 poles (-33.1443, -39.6532) (-33.0225, -39.6453) (-32.903, -39.6404) (-32.7841, -39.629) (-32.6853, -39.6195) (-32.6235, -39.5553) (-32.6159, -39.4653) (-32.6066, -39.3535) (-32.6453, -39.2828) (-32.7546, -39.2654) (-32.8913, -39.2438) (-33.0312, -39.2378) (-33.1699, -39.2352) (-33.2717, -39.2333) (-33.3755, -39.2384) (-33.4753, -39.2572) (-33.5813, -39.2771) (-33.6177, -39.3413) (-33.6151, -39.4584) (-33.6131, -39.5459) (-33.5626, -39.6128) (-33.4656, -39.6279) (-33.3593, -39.6445) (-33.2504, -39.6455) (-33.1443, -39.6532) knots 0 0 0 0 1 1 1 2 2 2 3 3 3 4 4 4 5 5 5 6 6 6 7 7 7 8 8 8 8
  line L372 (-33.1443, -39.6532) -> (-33.0225, -39.6453) construction
  line L373 (-33.0225, -39.6453) -> (-32.903, -39.6404) construction
  line L374 (-32.903, -39.6404) -> (-32.7841, -39.629) construction
  line L375 (-32.7841, -39.629) -> (-32.6853, -39.6195) construction
  line L376 (-32.6853, -39.6195) -> (-32.6235, -39.5553) construction
  line L377 (-32.6235, -39.5553) -> (-32.6159, -39.4653) construction
  line L378 (-32.6159, -39.4653) -> (-32.6066, -39.3535) construction
  line L379 (-32.6066, -39.3535) -> (-32.6453, -39.2828) construction
  line L380 (-32.6453, -39.2828) -> (-32.7546, -39.2654) construction
  line L381 (-32.7546, -39.2654) -> (-32.8913, -39.2438) construction
  line L382 (-32.8913, -39.2438) -> (-33.0312, -39.2378) construction
  line L383 (-33.0312, -39.2378) -> (-33.1699, -39.2352) construction
  line L384 (-33.1699, -39.2352) -> (-33.2717, -39.2333) construction
  line L385 (-33.2717, -39.2333) -> (-33.3755, -39.2384) construction
  line L386 (-33.3755, -39.2384) -> (-33.4753, -39.2572) construction
  line L387 (-33.4753, -39.2572) -> (-33.5813, -39.2771) construction
  line L388 (-33.5813, -39.2771) -> (-33.6177, -39.3413) construction
  line L389 (-33.6177, -39.3413) -> (-33.6151, -39.4584) construction
  line L390 (-33.6151, -39.4584) -> (-33.6131, -39.5459) construction
  line L391 (-33.6131, -39.5459) -> (-33.5626, -39.6128) construction
  line L392 (-33.5626, -39.6128) -> (-33.4656, -39.6279) construction
  line L393 (-33.4656, -39.6279) -> (-33.3593, -39.6445) construction
  line L394 (-33.3593, -39.6445) -> (-33.2504, -39.6455) construction
  line L395 (-33.2504, -39.6455) -> (-33.1443, -39.6532) construction
  spline S13 degree 3 poles (-33.7218, -35.9729) (-33.7218, -35.7863) (-33.7218, -35.6014) (-33.7218, -35.4122) (-33.6813, -35.4122) (-33.645, -35.4122) (-33.6007, -35.4122) (-33.6007, -35.5512) (-33.6007, -35.6879) (-33.6007, -35.8305) (-33.4656, -35.8305) (-33.3384, -35.8305) (-33.2035, -35.8305) (-33.2035, -35.702) (-33.2035, -35.5771) (-33.2035, -35.4457) (-33.1549, -35.4457) (-33.1139, -35.4457) (-33.0645, -35.4457) (-33.0645, -35.5708) (-33.0645, -35.6959) (-33.0645, -35.8287) (-32.924, -35.8287) (-32.7915, -35.8287) (-32.6493, -35.8287) (-32.6493, -35.686) (-32.6493, -35.5441) (-32.6493, -35.3972) (-32.604, -35.3972) (-32.5681, -35.3972) (-32.5249, -35.3972) (-32.5249, -35.5874) (-32.5249, -35.7773) (-32.5249, -35.9729) (-32.9229, -35.9729) (-33.3195, -35.9729) (-33.7218, -35.9729) knots 0 0 0 0 1 1 1 2 2 2 3 3 3 4 4 4 5 5 5 6 6 6 7 7 7 8 8 8 9 9 9 10 10 10 11 11 11 12 12 12 12
  line L396 (-33.7218, -35.9729) -> (-33.7218, -35.7863) construction
  line L397 (-33.7218, -35.7863) -> (-33.7218, -35.6014) construction
  line L398 (-33.7218, -35.6014) -> (-33.7218, -35.4122) construction
  line L399 (-33.7218, -35.4122) -> (-33.6813, -35.4122) construction
  line L400 (-33.6813, -35.4122) -> (-33.645, -35.4122) construction
  line L401 (-33.645, -35.4122) -> (-33.6007, -35.4122) construction
  line L402 (-33.6007, -35.4122) -> (-33.6007, -35.5512) construction
  line L403 (-33.6007, -35.5512) -> (-33.6007, -35.6879) construction
  line L404 (-33.6007, -35.6879) -> (-33.6007, -35.8305) construction
  line L405 (-33.6007, -35.8305) -> (-33.4656, -35.8305) construction
  line L406 (-33.4656, -35.8305) -> (-33.3384, -35.8305) construction
  line L407 (-33.3384, -35.8305) -> (-33.2035, -35.8305) construction
  line L408 (-33.2035, -35.8305) -> (-33.2035, -35.702) construction
  line L409 (-33.2035, -35.702) -> (-33.2035, -35.5771) construction
  line L410 (-33.2035, -35.5771) -> (-33.2035, -35.4457) construction
  line L411 (-33.2035, -35.4457) -> (-33.1549, -35.4457) construction
  line L412 (-33.1549, -35.4457) -> (-33.1139, -35.4457) construction
  line L413 (-33.1139, -35.4457) -> (-33.0645, -35.4457) construction
  line L414 (-33.0645, -35.4457) -> (-33.0645, -35.5708) construction
  line L415 (-33.0645, -35.5708) -> (-33.0645, -35.6959) construction
  line L416 (-33.0645, -35.6959) -> (-33.0645, -35.8287) construction
  line L417 (-33.0645, -35.8287) -> (-32.924, -35.8287) construction
  line L418 (-32.924, -35.8287) -> (-32.7915, -35.8287) construction
  line L419 (-32.7915, -35.8287) -> (-32.6493, -35.8287) construction
  line L420 (-32.6493, -35.8287) -> (-32.6493, -35.686) construction
  line L421 (-32.6493, -35.686) -> (-32.6493, -35.5441) construction
  line L422 (-32.6493, -35.5441) -> (-32.6493, -35.3972) construction
  line L423 (-32.6493, -35.3972) -> (-32.604, -35.3972) construction
  line L424 (-32.604, -35.3972) -> (-32.5681, -35.3972) construction
  line L425 (-32.5681, -35.3972) -> (-32.5249, -35.3972) construction
  line L426 (-32.5249, -35.3972) -> (-32.5249, -35.5874) construction
  line L427 (-32.5249, -35.5874) -> (-32.5249, -35.7773) construction
  line L428 (-32.5249, -35.7773) -> (-32.5249, -35.9729) construction
  line L429 (-32.5249, -35.9729) -> (-32.9229, -35.9729) construction
  line L430 (-32.9229, -35.9729) -> (-33.3195, -35.9729) construction
  line L431 (-33.3195, -35.9729) -> (-33.7218, -35.9729) construction
  spline S14 degree 3 poles (-32.5221, -36.967) (-32.5221, -37.1541) (-32.5221, -37.3365) (-32.5221, -37.5261) (-32.9215, -37.5261) (-33.3182, -37.5261) (-33.7211, -37.5261) (-33.7211, -37.3469) (-33.7211, -37.1678) (-33.7211, -36.9834) (-33.6838, -36.9834) (-33.6478, -36.9834) (-33.602, -36.9834) (-33.602, -37.1145) (-33.602, -37.2476) (-33.602, -37.3859) (-33.4653, -37.3859) (-33.3382, -37.3859) (-33.2044, -37.3859) (-33.2044, -37.2582) (-33.2044, -37.133) (-33.2044, -37.0014) (-33.1569, -37.0014) (-33.1156, -37.0014) (-33.0639, -37.0014) (-33.0639, -37.1259) (-33.0639, -37.2532) (-33.0639, -37.3858) (-32.9233, -37.3858) (-32.7927, -37.3858) (-32.6512, -37.3858) (-32.6512, -37.2492) (-32.6512, -37.1106) (-32.6512, -36.967) (-32.6044, -36.967) (-32.5685, -36.967) (-32.5221, -36.967) knots 0 0 0 0 1 1 1 2 2 2 3 3 3 4 4 4 5 5 5 6 6 6 7 7 7 8 8 8 9 9 9 10 10 10 11 11 11 12 12 12 12
  line L432 (-32.5221, -36.967) -> (-32.5221, -37.1541) construction
  line L433 (-32.5221, -37.1541) -> (-32.5221, -37.3365) construction
  line L434 (-32.5221, -37.3365) -> (-32.5221, -37.5261) construction
  line L435 (-32.5221, -37.5261) -> (-32.9215, -37.5261) construction
  line L436 (-32.9215, -37.5261) -> (-33.3182, -37.5261) construction
  line L437 (-33.3182, -37.5261) -> (-33.7211, -37.5261) construction
  line L438 (-33.7211, -37.5261) -> (-33.7211, -37.3469) construction
  line L439 (-33.7211, -37.3469) -> (-33.7211, -37.1678) construction
  line L440 (-33.7211, -37.1678) -> (-33.7211, -36.9834) construction
  line L441 (-33.7211, -36.9834) -> (-33.6838, -36.9834) construction
  line L442 (-33.6838, -36.9834) -> (-33.6478, -36.9834) construction
  line L443 (-33.6478, -36.9834) -> (-33.602, -36.9834) construction
  line L444 (-33.602, -36.9834) -> (-33.602, -37.1145) construction
  line L445 (-33.602, -37.1145) -> (-33.602, -37.2476) construction
  line L446 (-33.602, -37.2476) -> (-33.602, -37.3859) construction
  line L447 (-33.602, -37.3859) -> (-33.4653, -37.3859) construction
  line L448 (-33.4653, -37.3859) -> (-33.3382, -37.3859) construction
  line L449 (-33.3382, -37.3859) -> (-33.2044, -37.3859) construction
  line L450 (-33.2044, -37.3859) -> (-33.2044, -37.2582) construction
  line L451 (-33.2044, -37.2582) -> (-33.2044, -37.133) construction
  line L452 (-33.2044, -37.133) -> (-33.2044, -37.0014) construction
  line L453 (-33.2044, -37.0014) -> (-33.1569, -37.0014) construction
  line L454 (-33.1569, -37.0014) -> (-33.1156, -37.0014) construction
  line L455 (-33.1156, -37.0014) -> (-33.0639, -37.0014) construction
  line L456 (-33.0639, -37.0014) -> (-33.0639, -37.1259) construction
  line L457 (-33.0639, -37.1259) -> (-33.0639, -37.2532) construction
  line L458 (-33.0639, -37.2532) -> (-33.0639, -37.3858) construction
  line L459 (-33.0639, -37.3858) -> (-32.9233, -37.3858) construction
  line L460 (-32.9233, -37.3858) -> (-32.7927, -37.3858) construction
  line L461 (-32.7927, -37.3858) -> (-32.6512, -37.3858) construction
  line L462 (-32.6512, -37.3858) -> (-32.6512, -37.2492) construction
  line L463 (-32.6512, -37.2492) -> (-32.6512, -37.1106) construction
  line L464 (-32.6512, -37.1106) -> (-32.6512, -36.967) construction
  line L465 (-32.6512, -36.967) -> (-32.6044, -36.967) construction
  line L466 (-32.6044, -36.967) -> (-32.5685, -36.967) construction
  line L467 (-32.5685, -36.967) -> (-32.5221, -36.967) construction
  spline S15 degree 3 poles (-33.0448, -40.4532) (-32.8678, -40.4532) (-32.6998, -40.4532) (-32.5249, -40.4532) (-32.5249, -40.4951) (-32.5249, -40.5305) (-32.5249, -40.5744) (-32.9214, -40.5744) (-33.3194, -40.5744) (-33.7337, -40.5744) (-33.7262, -40.4326) (-33.7249, -40.2932) (-33.7081, -40.1556) (-33.7026, -40.1104) (-33.6663, -40.0579) (-33.6285, -40.0296) (-33.5095, -39.9405) (-33.3719, -39.942) (-33.2369, -39.9842) (-33.0921, -40.0293) (-33.0529, -40.1502) (-33.0453, -40.286) (-33.0424, -40.3372) (-33.0448, -40.3888) (-33.0448, -40.4532) knots 0 0 0 0 1 1 1 2 2 2 3 3 3 4 4 4 5 5 5 6 6 6 7 7 7 8 8 8 8
  line L468 (-33.0448, -40.4532) -> (-32.8678, -40.4532) construction
  line L469 (-32.8678, -40.4532) -> (-32.6998, -40.4532) construction
  line L470 (-32.6998, -40.4532) -> (-32.5249, -40.4532) construction
  line L471 (-32.5249, -40.4532) -> (-32.5249, -40.4951) construction
  line L472 (-32.5249, -40.4951) -> (-32.5249, -40.5305) construction
  line L473 (-32.5249, -40.5305) -> (-32.5249, -40.5744) construction
  line L474 (-32.5249, -40.5744) -> (-32.9214, -40.5744) construction
  line L475 (-32.9214, -40.5744) -> (-33.3194, -40.5744) construction
  line L476 (-33.3194, -40.5744) -> (-33.7337, -40.5744) construction
  line L477 (-33.7337, -40.5744) -> (-33.7262, -40.4326) construction
  line L478 (-33.7262, -40.4326) -> (-33.7249, -40.2932) construction
  line L479 (-33.7249, -40.2932) -> (-33.7081, -40.1556) construction
  line L480 (-33.7081, -40.1556) -> (-33.7026, -40.1104) construction
  line L481 (-33.7026, -40.1104) -> (-33.6663, -40.0579) construction
  line L482 (-33.6663, -40.0579) -> (-33.6285, -40.0296) construction
  line L483 (-33.6285, -40.0296) -> (-33.5095, -39.9405) construction
  line L484 (-33.5095, -39.9405) -> (-33.3719, -39.942) construction
  line L485 (-33.3719, -39.942) -> (-33.2369, -39.9842) construction
  line L486 (-33.2369, -39.9842) -> (-33.0921, -40.0293) construction
  line L487 (-33.0921, -40.0293) -> (-33.0529, -40.1502) construction
  line L488 (-33.0529, -40.1502) -> (-33.0453, -40.286) construction
  line L489 (-33.0453, -40.286) -> (-33.0424, -40.3372) construction
  line L490 (-33.0424, -40.3372) -> (-33.0448, -40.3888) construction
  line L491 (-33.0448, -40.3888) -> (-33.0448, -40.4532) construction
  spline S16 degree 3 poles (-33.1897, -40.4513) (-33.1753, -40.2316) (-33.1873, -40.1626) (-33.2636, -40.1303) (-33.3524, -40.0926) (-33.4497, -40.0844) (-33.5317, -40.1447) (-33.6425, -40.2261) (-33.5858, -40.3452) (-33.5977, -40.4513) (-33.4554, -40.4513) (-33.3252, -40.4513) (-33.1897, -40.4513) knots 0 0 0 0 1 1 1 2 2 2 3 3 3 4 4 4 4
  line L492 (-33.1897, -40.4513) -> (-33.1753, -40.2316) construction
  line L493 (-33.1753, -40.2316) -> (-33.1873, -40.1626) construction
  line L494 (-33.1873, -40.1626) -> (-33.2636, -40.1303) construction
  line L495 (-33.2636, -40.1303) -> (-33.3524, -40.0926) construction
  line L496 (-33.3524, -40.0926) -> (-33.4497, -40.0844) construction
  line L497 (-33.4497, -40.0844) -> (-33.5317, -40.1447) construction
  line L498 (-33.5317, -40.1447) -> (-33.6425, -40.2261) construction
  line L499 (-33.6425, -40.2261) -> (-33.5858, -40.3452) construction
  line L500 (-33.5858, -40.3452) -> (-33.5977, -40.4513) construction
  line L501 (-33.5977, -40.4513) -> (-33.4554, -40.4513) construction
  line L502 (-33.4554, -40.4513) -> (-33.3252, -40.4513) construction
  line L503 (-33.3252, -40.4513) -> (-33.1897, -40.4513) construction
  point P0 (0, 0)
  constraints: 30 other
extrude "Extrusion3" cut sketch "Sketch2" against normal blind 0.5 contours S0 | S1 | S2 | S3 | S5 | S6 | S7 | S9 | S11 | S13 | S14 | S15